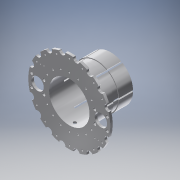
# Autodesk Inventor part: Fixture
Saved by Autodesk Inventor 2016 (Build 200138000, 138)
## iProperties
Created: 2015-07-19
Part Number: Fixture
Material: Generic
Document SubType Name: Modeling
Designer: bastli
Density: 1 g/cm^3
Appearance: Aluminum - Polished
nema_11_cutout: 23,000 mm
cup_big_radius: 74,000 mm
cup_small_radius: 66,000 mm
nema_11_transmission_radius: 5,300 mm
nema_11_transmission_length: 20,000 mm
nema_11_transmission_foot: 2,000 mm
nema_11_transmission_cut_diameter: 4,650 mm
transmission_diameter: 50,900 mm
stand_height: 4,500 mm
nema_11_transmission_cut_length: 14,750 mm
nema_11_foot_diameter: 22,000 mm
nema_11_width: 28,300 mm
nema_11_hole_distance: 23,000 mm
nema_11_length: 51,000 mm
thickness: 3,000 mm
outer_radius: 151,200 mm
pvc_radius: 76,600 mm
fixture_height: 72,000 mm
height: 12,100 mm
stepper_center_distance: 58,450 mm
Author: bastli
Autodesk Inventor part; units mm, degrees
ref_plane "YZ Plane" through (0, 0, 0) normal (1, 0, 0) x (0, 1, 0)
sketch "Sketch1" plane through (0, 0, 0) normal (0, 1, 0) x (-1, 0, 0)
  circle A0 centre (0, 0) radius 75.6
  circle A1 centre (0, 0) radius 38.3
  circle A2 centre (0, 0) radius 41.3
  circle A3 centre (0, 0) radius 37.3
  line L0 (75.6, 0) -> (-75.6, 0) construction
  line L1 (0, 75.6) -> (0, -75.6) construction
  line L2 (69.95, -11.5) -> (46.95, -11.5) construction
  line L3 (46.95, -11.5) -> (46.95, 11.5) construction
  line L4 (46.95, 11.5) -> (69.95, 11.5) construction
  line L5 (69.95, 11.5) -> (69.95, -11.5) construction
  line L6 (69.95, -11.5) -> (46.95, 11.5) construction
  line L7 (46.95, -11.5) -> (69.95, 11.5) construction
  line L8 (72.6, -14.15) -> (44.3, -14.15) construction
  line L9 (44.3, -14.15) -> (44.3, 14.15) construction
  line L10 (44.3, 14.15) -> (72.6, 14.15) construction
  line L11 (72.6, 14.15) -> (72.6, -14.15) construction
  line L12 (72.6, -14.15) -> (44.3, 14.15) construction
  line L13 (44.3, -14.15) -> (72.6, 14.15) construction
  line L14 (72.6, 0) -> (75.6, 0) construction
  line L15 (44.3, 0) -> (41.3, 0) construction
  circle A4 centre (58.45, 0) radius 11.5
  circle A5 centre (-58.45, 0) radius 11.5
  point P0 (-69.95, 11.5)
  point P1 (-46.95, 11.5)
  point P2 (-46.95, -11.5)
  point P3 (-69.95, -11.5)
  dimension "d0" = 151.2
  dimension "d1" = 76.6
  dimension "d2" = 3
  dimension "d3" = 74.6
  dimension "d4" = 23
  dimension "d5" = 23
  dimension "d6" = 28.3
  dimension "d7" = 28.3
  dimension "d30" = 23
  constraints: 32 end point, 9 midpoint, 8 coincident, 5 centre point, 5 symmetric about line, 4 parallel, 4 point on circle, 3 horizontal, 2 collinear, 2 perpendicular, 2 point on line, 1 horizontal alignment, 1 vertical, 3 other
  measures "d0" diameter of A0
  measures "d1" diameter of A1
  measures "d3" diameter of A3
  measures "d4" distance of L3.end L4.end
  measures "d5" distance of L4.end L2.start
  measures "d6" distance of L9.end L10.end
  measures "d7" distance of L10.end L8.start
  measures "d30" diameter of A4
extrude "Extrusion1" add sketch "Sketch1" against normal blind 4.5 contours A0 | A1 | A2 | A4 | A5
extrude "Extrusion2" add sketch "Sketch1" along normal blind 72 contours A2
ref_plane "Work Plane1" through (0, 36, 0) normal (0, 1, 0) x (1, 0, 0)
sketch "Sketch2" plane through (0, 36, 0) normal (0, 1, 0) x (1, 0, 0)
  circle A0 centre (0, 0) radius 38.3 projected
  circle A1 centre (0, 0) radius 41.3 projected
  circle A2 centre (0, 0) radius 39.8
  dimension "d14" = 1.5
  constraints: 1 centre point
  measures "d14" radial gap between concentric circles of A1 A2
extrude "Extrusion3" cut sketch "Sketch2" along normal blind 10 contours A1
sketch "Sketch3" plane through (0, 72, 0) normal (0, 1, 0) x (1, 0, 0)
  circle A0 centre (0, 0) radius 41.3 projected
  circle A1 centre (0, 0) radius 38.3 projected
  line L0 (0, 0) -> (41.3, 0) construction
  line L1 (0, 0) -> (41.2748, 1.4413) construction
  circle A2 centre (0, 0) radius 41.3 projected
  line L2 (0, 0) -> (41.2748, -1.4413) construction
  line L3 (41.2748, 1.4413) -> (38.2767, 1.3367)
  circle A3 centre (0, 0) radius 38.3 projected
  line L4 (41.2748, -1.4413) -> (38.2767, -1.3367)
  dimension "d17" = 4
  constraints: 10 end point, 7 point on circle, 2 point on line, 1 horizontal, 1 other
  measures "d17" angle of L2 L1
extrude "Extrusion4" cut sketch "Sketch3" against normal blind 48 contours A0 L4 A1 L3 picked at (40.2991, -0.1602)
pattern_circular "Circular Pattern1" count 6 over 360 about axis through (0, 0, 0) along (0, 1, 0) of "Extrusion4"
fillet "Fillet1" radius 3 1 edges at (41.3, 0, 0)
hole "Hole1" at (-69.95, 0, 11.5) at (-46.95, 0, 11.5) at (-46.95, 0, -11.5) at (-69.95, 0, -11.5) at (69.95, 0, 11.5) at (46.95, 0, 11.5) at (46.95, 0, -11.5) at (69.95, 0, -11.5) direction (0, -1, 0) diameter 2.6 end through all
extrude "Extrusion5" cut sketch "Sketch1" against normal through all contours A4 | A5
sketch "Sketch4" plane through (0, -4.5, 0) normal (0, -1, 0) x (1, 0, 0)
  circle A0 centre (-46.95, -11.5) radius 1.3 construction
  circle A1 centre (-69.95, 11.5) radius 1.3 construction
  circle A2 centre (-46.95, 11.5) radius 1.3 construction
  circle A3 centre (46.95, 11.5) radius 1.3 construction
  circle A4 centre (46.95, -11.5) radius 1.3 construction
  circle A5 centre (69.95, -11.5) radius 1.3 construction
  circle A6 centre (69.95, 11.5) radius 1.3 construction
  circle A7 centre (-69.95, -11.5) radius 1.3 construction
  point P0 (0, 0)
  constraints: 8 coincident
hole "Hole2" at (-69.95, -4.5, 11.5) at (-46.95, -4.5, 11.5) at (-46.95, -4.5, -11.5) at (-69.95, -4.5, -11.5) at (46.95, -4.5, -11.5) at (46.95, -4.5, 11.5) at (69.95, -4.5, 11.5) at (69.95, -4.5, -11.5) direction (0, 1, 0) diameter 5.4 depth 3 tip angle 118
sketch "Sketch5" plane through (0, 0, 0) normal (0, 1, 0) x (1, 0, 0)
  circle A0 centre (-58.45, 0) radius 11.5 construction
  circle A1 centre (58.45, 0) radius 11.5 construction
  circle A2 centre (46.95, 11.5) radius 1.3 construction
  circle A3 centre (69.95, -11.5) radius 1.3 construction
  circle A4 centre (-46.95, 11.5) radius 1.3 construction
  circle A5 centre (-69.95, -11.5) radius 1.3 construction
  circle A6 centre (-46.95, -11.5) radius 1.3 construction
  circle A7 centre (-69.95, 11.5) radius 1.3 construction
  circle A8 centre (46.95, -11.5) radius 1.3 construction
  circle A9 centre (69.95, 11.5) radius 1.3 construction
  circle A10 centre (0, 0) radius 75.6 construction
  circle A11 centre (0, 0) radius 44.3 construction
  circle A12 centre (0, 0) radius 69.6 construction
  circle A13 centre (0, 0) radius 47.3 construction
  line L0 (0, -47.3) -> (0, -69.6) construction
  line L1 (0, -47.3) -> (0, 0) construction
  circle A14 centre (58.45, 0) radius 11.5 projected
  circle A15 centre (0, 0) radius 44.3 projected
  line L2 (58.45, 0) -> (0, 0) construction
  point P0 (23.8046, -65.4026)
  point P1 (16.1776, -44.4475)
  point P2 (44.738, -53.3167)
  point P3 (30.4039, -36.2339)
  point P4 (60.2754, -34.8)
  point P5 (40.963, -23.65)
  point P6 (-16.1776, -44.4475)
  point P7 (-23.8046, -65.4026)
  point P8 (-30.4039, -36.2339)
  point P9 (-44.738, -53.3167)
  point P10 (-40.963, -23.65)
  point P11 (-60.2754, -34.8)
  point P12 (0, 69.6)
  point P13 (0, 47.3)
  point P14 (23.8046, 65.4026)
  point P15 (16.1776, 44.4475)
  point P16 (44.738, 53.3167)
  point P17 (30.4039, 36.2339)
  point P18 (60.2754, 34.8)
  point P19 (40.963, 23.65)
  point P20 (-16.1776, 44.4475)
  point P21 (-23.8046, 65.4026)
  point P22 (-30.4039, 36.2339)
  point P23 (-44.738, 53.3167)
  point P24 (-40.963, 23.65)
  point P25 (-60.2754, 34.8)
  dimension "d40" = 6
  dimension "d41" = 3
  dimension "d44" = 60
  dimension "d48" = 60
  constraints: 14 symmetric about line, 6 end point, 2 vertical, 2 vertical alignment, 1 horizontal, 18 other
hole "Hole3" at (0, 0, 69.6) at (0, 0, 47.3) at (23.8046, 0, 65.4026) at (16.1776, 0, 44.4475) at (44.738, 0, 53.3167) at (30.4039, 0, 36.2339) at (60.2754, 0, 34.8) at (40.963, 0, 23.65) at (-16.1776, 0, 44.4475) at (-23.8046, 0, 65.4026) at (-30.4039, 0, 36.2339) at (-44.738, 0, 53.3167) at (-40.963, 0, 23.65) at (-60.2754, 0, 34.8) at (40.963, 0, -23.65) at (60.2754, 0, -34.8) at (44.738, 0, -53.3167) at (30.4039, 0, -36.2339) at (16.1776, 0, -44.4475) at (23.8046, 0, -65.4026) at (0, 0, -47.3) at (0, 0, -69.6) at (-23.8046, 0, -65.4026) at (-16.1776, 0, -44.4475) at (-30.4039, 0, -36.2339) at (-44.738, 0, -53.3167) at (-40.963, 0, -23.65) at (-60.2754, 0, -34.8) direction (0, -1, 0) diameter 3.1 end through all
ref_plane "Work Plane2" through (0, 0, -41.3) normal (0, 0, 1) x (1, 0, 0)
sketch "Sketch6" plane through (0, 0, -41.3) normal (0, 0, 1) x (1, 0, 0)
  line L0 (0, 0) -> (0, 6) construction
  dimension "d57" = 6
  constraints: 2 end point, 1 vertical
  measures "d57" distance of L0.start L0.end
hole "Hole4" at (0, 6, -41.3) direction (0, 0, 1) diameter 6 end through all
sketch "Sketch7" plane through (0, 0, 0) normal (0, 1, 0) x (1, 0, 0)
  circle A0 centre (0, 0) radius 75.6 projected
  circle A1 centre (13.1278, -74.4515) radius 6
  line L0 (0, 0) -> (0, -75.6) construction
  line L1 (13.1278, -74.4515) -> (0, 0) construction
  dimension "d65" = 12
  dimension "d66" = 10
  constraints: 4 end point, 2 point on circle, 1 centre point, 1 vertical
  measures "d65" diameter of A1
  measures "d66" angle of L0 L1
extrude "Extrusion6" cut sketch "Sketch7" against normal up to surface (4.5 mm away) contours A1 A0 | A0 A1 picked at (12.5484, -72.5189) picked at (13.4888, -76.4007)
pattern_circular "Circular Pattern2" count 4 over 60 about axis through (0, 0, 0) along (0, 1, 0) of "Extrusion6"
mirror "Mirror2" about plane through (0, 0, 0) normal (1, 0, 0) of "Extrusion6", "Circular Pattern2"
mirror "Mirror3" about plane through (0, 0, 0) normal (0, 0, 1) of "Extrusion6", "Circular Pattern2", "Mirror2"
sketch "Sketch10" plane through (0, -4.5, 0) normal (0, -1, 0) x (1, 0, 0)
  circle A0 centre (0, 0) radius 37.3 projected
  circle A1 centre (58.45, 0) radius 11.5 projected
  circle A2 centre (0, 0) radius 33 construction
  circle A3 centre (58.45, 0) radius 25.45 construction
  dimension "stepper_center_distance" = 58.45
  dimension "stepper_hole_size" = 23
  dimension "d97" = 66
  dimension "transmission_diameter" = 50.9
  constraints: 2 centre point, 2 coincident, 1 tangent
  measures "stepper_center_distance" distance of A1.centre point (0, 0)
  measures "stepper_hole_size" diameter of A1
  measures "d97" diameter of A2
  measures "transmission_diameter" diameter of A3
sketch "Sketch9" plane through (0, -4.5, 0) normal (0, -1, 0) x (1, 0, 0)
  line L0 (60.9405, -25.3278) -> (43.0269, -27.0893)
  line L1 (43.0269, -27.0893) -> (43.3205, -30.0749)
  line L2 (43.3205, -30.0749) -> (61.2341, -28.3134)
  line L3 (61.2341, -28.3134) -> (60.9405, -25.3278)
  line L4 (43.3205, -30.0749) -> (56.0591, -28.8223)
  line L5 (56.0591, -28.8223) -> (56.6952, -35.2911)
  line L6 (56.6952, -35.2911) -> (43.9566, -36.5437)
  line L7 (43.9566, -36.5437) -> (43.3205, -30.0749)
  line L8 (43.9566, -36.5437) -> (56.6952, -35.2911)
  line L9 (56.6952, -35.2911) -> (57.0181, -38.5753)
  line L10 (57.0181, -38.5753) -> (44.2795, -39.8279)
  line L11 (44.2795, -39.8279) -> (43.9566, -36.5437)
  arc A0 (72.8675, -20.1416) -> (68.7665, -31.409) centre (71.0408, -25.8567) ccw construction
  line L12 (49.6898, -29.4486) -> (50.3259, -35.9174) construction
  circle A1 centre (58.45, 0) radius 11.5 construction
  circle A2 centre (58.45, 0) radius 25.45 construction
  point P0 (46.9447, -34.7427)
  point P1 (53.4135, -34.1066)
  dimension "d74" = 18
  dimension "d76" = 6.5
  dimension "d78" = 9.5
  dimension "d79" = 12.8
  dimension "d80" = 3.3
  dimension "d81" = 4
  dimension "d82" = 1.5
  dimension "d83" = 6.5
  dimension "d99" = 50.9
  constraints: 26 end point, 6 parallel, 3 perpendicular, 2 midpoint, 1 centre point, 1 coincident, 1 line through centre, 1 point on line, 1 symmetric about line, 1 tangent
  measures "d74" distance of L0.start L0.end
  measures "d76" distance of L6.end L1.end
  measures "d78" distance between parallel lines of L6 L0
  measures "d79" distance between parallel lines of L7 L5
  measures "d80" distance between parallel lines of L6 L10
  measures "d81" distance edge to line of A0 L3
  measures "d82" distance from line of L6 point (46.945, -34.743)
  measures "d83" distance of point (53.413, -34.107) point (46.945, -34.743)
  measures "d99" diameter of A2
hole "Hole5" at (46.9447, -4.5, -34.7427) at (53.4135, -4.5, -34.1066) direction (0, 1, 0) diameter 2.1 end through all
pattern_circular "Circular Pattern3" count 2 over 360 about axis through (0, 0, 0) along (0, -1, 0) of "Hole5"
equation "\"d0\" = outer_radius"
equation "\"d1\" = pvc_radius"
equation "\"d2\" = thickness"
equation "\"d3\" = pcv_foot_radius"
equation "\"d4\" = nema_11_hole_distance"
equation "\"d5\" = nema_11_hole_distance"
equation "\"d6\" = nema_11_width"
equation "\"d7\" = nema_11_width"
equation "\"d30\" = nema_11_cutout"
equation "\"d8\" = stand_height"
equation "\"d10\" = fixture_height"
equation "\"d14\" = 0.5 * thickness"
equation "\"d18\" = 16 * thickness"
equation "\"d38\" = thickness"
equation "\"d40\" = 2 * thickness"
equation "\"d41\" = thickness"
equation "\"d57\" = 2 * thickness"
equation "\"d97\" = cup_small_radius"
equation "\"d99\" = transmission_diameter"
equation "\"thickness\" = 3"
equation "\"outer_radius\" = 6 * thickness + pvc_radius + 2 * nema_11_width"
equation "\"pvc_radius\" = 76.6"
equation "\"pcv_foot_radius\" = 74.6"
equation "\"nema_11_width\" = 28.3"
equation "\"nema_11_hole_distance\" = 23"
equation "\"fixture_height\" = 24 * thickness"
equation "\"d13\" = 0.5 * fixture_height"
equation "\"m3_through\" = 3.4"
equation "\"m3_head\" = 6"
equation "\"m3_hold\" = 3.1"
equation "\"height\" = 12.1"
equation "\"cup_big_radius\" = 74"
equation "\"cup_small_radius\" = 66"
equation "\"nema_11_transmission_radius\" = 5.3"
equation "\"nema_11_transmission_length\" = 20"
equation "\"nema_11_transmission_foot\" = 2"
equation "\"nema_11_transmission_cut_diameter\" = 4.65"
equation "\"stand_height\" = 1.5 * thickness"
equation "\"nema_11_transmission_cut_length\" = 14.75"
equation "\"nema_11_foot_diameter\" = 22"
equation "\"nema_11_length\" = 51"
equation "\"nema_11_cutout\" = 23"
body "Solid1"
